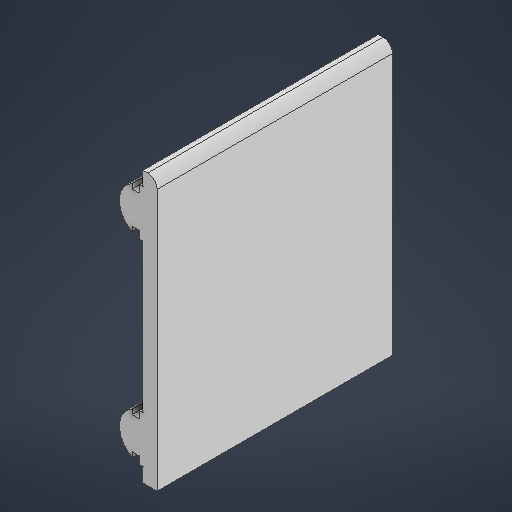
# Autodesk Inventor part: Cover of Sensors
Saved by Autodesk Inventor 2026.2 (Build 302298010, 298A)
## iProperties
Created: 2026-05-05
Part Number: Cover of Sensors
Material: Generic
Document SubType Name: Modeling
Designer: lenovo
Density: 1 g/cm^3
Appearance: Default
Author: lenovo
Autodesk Inventor part; units mm, degrees
ref_plane "YZ Plane" through (0, 0, 0) normal (1, 0, 0) x (0, 1, 0)
ref_plane "XZ Plane" through (0, 0, 0) normal (0, 1, 0) x (-1, 0, 0)
ref_plane "XY Plane" through (0, 0, 0) normal (0, 0, 1) x (1, 0, 0)
sketch "Sketch1" plane through (0, 0, 0) normal (1, 0, 0) x (0, 1, 0)
  line L0 (-28.75, 25) -> (28.75, 25)
  line L1 (28.75, 25) -> (28.75, -25)
  line L2 (28.75, -25) -> (-28.75, -25)
  line L3 (-28.75, -25) -> (-28.75, 25)
  line L4 (-28.75, 25) -> (28.75, -25) construction
  line L5 (28.75, 25) -> (-28.75, -25) construction
  point P0 (0, 0)
  dimension "d0" = 57.5
  dimension "d1" = 50
  constraints: 12 end point, 2 midpoint, 2 parallel, 1 horizontal, 1 perpendicular
  measures "d0" distance of L1.end L2.end
  measures "d1" distance of L0.end L1.end
extrude "Extrusion1" add sketch "Sketch1" along normal blind 3
sketch "Sketch4" plane through (0, -28.75, 25) normal (0, 0, 1) x (1, 0, 0)
  line L0 (0, 0) -> (0, 57.5) projected
  arc A0 (0, 54.5) -> (0, 44.5) centre (0, 49.5) ccw
  line L1 (-0.8, 44.5644) -> (-0.8, 46.0644)
  line L2 (-0.8, 46.0644) -> (-2.3, 46.0644)
  line L3 (-2.3, 46.0644) -> (-2.3, 45.0604)
  line L4 (-5, 49.5) -> (0, 49.5) construction
  line L5 (-0.8, 54.4356) -> (-0.8, 52.9356)
  line L6 (-0.8, 52.9356) -> (-2.3, 52.9356)
  line L7 (-2.3, 52.9356) -> (-2.3, 53.9396)
  line L8 (0, 0) -> (3, 0) projected
  arc A1 (0, 13) -> (0, 3) centre (0, 8) ccw
  line L9 (-0.8, 3.0644) -> (-0.8, 4.5644)
  line L10 (-0.8, 4.5644) -> (-2.3, 4.5644)
  line L11 (-2.3, 4.5644) -> (-2.3, 3.5604)
  line L12 (-5, 8) -> (0, 8) construction
  line L13 (-0.8, 12.9356) -> (-0.8, 11.4356)
  line L14 (-0.8, 11.4356) -> (-2.3, 11.4356)
  line L15 (-2.3, 11.4356) -> (-2.3, 12.4396)
  point P0 (0, 28.75)
  point P1 (-2.3, 53.9396)
  dimension "d15" = 1.5
  dimension "d16" = 1.5
  dimension "d17" = 0.8
  dimension "d25" = 3
  dimension "d26" = 10
  dimension "d28" = 1.5
  dimension "d31" = 10
  dimension "d32" = 3
  dimension "d33" = 1.5
  constraints: 28 end point, 10 point on circle, 8 symmetric about line, 4 point on line, 3 perpendicular, 3 vertical, 2 centre point, 2 horizontal
  measures "d15" distance of L1.start L1.end
  measures "d16" distance of L1.end L2.end
  measures "d17" horizontal distance of A0.end L1.start
  measures "d25" distance of A0.start L0.end
  measures "d26" distance of A1.end A1.start
  measures "d28" distance of L9.start L9.end
  measures "d31" distance of A0.end A0.start
  measures "d32" distance of L0.start A1.end
  measures "d33" distance of L9.end L10.end
extrude "Extrusion3" add sketch "Sketch4" against normal blind 49 contours A0 L1 L2 L3 L7 L6 L5 L0
fillet "Fillet2" radius 2 1 edges at (3, 28.75, 0)
extrude "Extrusion4" add sketch "Sketch4" against normal blind 49 contours A1 L9 L10 L11 L15 L14 L13 L0
body "Solid1"
